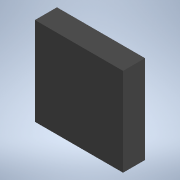
# Autodesk Inventor part: MPU_chip
Saved by Autodesk Inventor 2022 (Build 260153000, 153)
## iProperties
Created: 2022-03-19
Part Number: MPU_chip
Material: Generic
Document SubType Name: Modeling
Designer: dvorakj
Density: 1 g/cm^3
Appearance: Rubber - Black
Author: dvorakj
Autodesk Inventor part; units mm, degrees
ref_plane "YZ Plane" through (0, 0, 0) normal (1, 0, 0) x (0, 1, 0)
ref_plane "XZ Plane" through (0, 0, 0) normal (0, 1, 0) x (-1, 0, 0)
ref_plane "XY Plane" through (0, 0, 0) normal (0, 0, 1) x (1, 0, 0)
sketch "Sketch1" plane through (0, 0, 0) normal (0, 0, 1) x (1, 0, 0)
  line L0 (2, -12.1) -> (-2, -12.1)
  line L1 (-2, -12.1) -> (-2, -8.1)
  line L2 (-2, -8.1) -> (2, -8.1)
  line L3 (2, -8.1) -> (2, -12.1)
  line L4 (-12.5, -14.1) -> (12.5, -14.1) projected
  point P0 (0, 0)
  point P1 (0, -8.1)
  dimension "d0" = 4
  dimension "d1" = 4
  dimension "d2" = 2
  constraints: 8 end point, 2 parallel, 1 horizontal, 1 midpoint, 1 perpendicular, 1 vertical alignment
  measures "d0" distance of L1.end L2.end
  measures "d1" distance of L0.end L1.end
  measures "d2" distance between parallel lines of L4 L0
extrude "Extrusion1" add sketch "Sketch1" along normal blind 1
body "Solid1"
